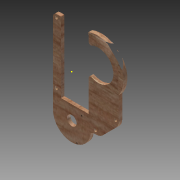
# Autodesk Inventor part: p1
Saved by Autodesk Inventor 2015 (Build 190159000, 159)
## iProperties
Created: 2016-02-03
Part Number: p1
Material: Generic
Document SubType Name: Modeling
Designer: david
Density: 1 g/cm^3
Appearance: Birch - Natural Polished
Author: david
Autodesk Inventor part; units mm, degrees
ref_plane "YZ Plane" through (0, 0, 0) normal (1, 0, 0) x (0, 1, 0)
ref_plane "XZ Plane" through (0, 0, 0) normal (0, 1, 0) x (-1, 0, 0)
ref_plane "XY Plane" through (0, 0, 0) normal (0, 0, 1) x (1, 0, 0)
sketch "Sketch1" plane through (0, 0, 0) normal (0, 1, 0) x (-1, 0, 0)
  line L0 (20, 45) -> (-20, 45)
  line L1 (-20, 45) -> (-20, -45)
  line L2 (-20, -45) -> (20, -45)
  line L3 (20, -45) -> (20, 45)
  line L4 (20, 45) -> (-20, -45) construction
  line L5 (-20, 45) -> (20, -45) construction
  arc A0 (-20, -45) -> (20, -45) centre (0, -45) ccw
  line L6 (20, -45) -> (20, -45)
  line L7 (20, -45) -> (20, 45)
  line L8 (20, 45) -> (20, 45)
  line L9 (20, 45) -> (20, -45)
  line L10 (-20, 45) -> (-50, 45)
  line L11 (-50, 45) -> (-50, -45)
  line L12 (-50, -45) -> (-20, -45)
  line L13 (-20, -45) -> (-20, 45)
  point P0 (0, 0)
  dimension "d0" = 40
  dimension "d1" = 90
  dimension "d7" = 0
  dimension "d8" = 90
  dimension "d35" = 30
  constraints: 28 end point, 6 equal length, 3 horizontal, 3 midpoint, 3 perpendicular, 2 point on circle, 1 centre point
  measures "d0" distance of L2.end L1.end
  measures "d1" distance of L1.end L0.end
  measures "d7" distance of L8.end L7.end
  measures "d8" distance of L7.end L6.end
  measures "d35" distance of L12.end L11.end
extrude "Extrusion1" add sketch "Sketch1" along normal blind 3.6
sketch "Sketch2" plane through (0, 3.6, 0) normal (0, 1, 0) x (1, 0, 0)
  arc A0 (20, 45) -> (-20, 45) centre (0, 45) ccw projected
  circle A1 centre (0, 45) radius 5.15
  point P0 (0, 0)
  dimension "d4" = 10.3
  constraints: 1 centre point, 1 coincident
  measures "d4" diameter of A1
extrude "Extrusion2" cut sketch "Sketch2" against normal blind 3.6
sketch "Sketch3" plane through (0, 0, 0) normal (0, -1, 0) x (1, 0, 0)
  line L0 (-20, 45) -> (50, 45) projected
  line L1 (-11.5, 45) -> (18, 45)
  line L2 (18, 45) -> (18, -30)
  line L3 (18, -30) -> (-11.5, -30)
  line L4 (-11.5, -30) -> (-11.5, 45)
  circle A0 centre (28, 20) radius 16.25
  line L5 (-20, -45) -> (-20, 45) projected
  line L6 (50, 45) -> (50, -45) projected
  point P0 (0, 0)
  point P1 (16, 45)
  dimension "d10" = 29.5
  dimension "d11" = 75
  dimension "d13" = 32.5
  dimension "d15" = 25
  dimension "d37" = 32
  dimension "d39" = 22
  constraints: 8 end point, 2 parallel, 1 centre point, 1 horizontal, 1 perpendicular, 1 point on line
  measures "d10" distance of L2.end L3.end
  measures "d11" distance of L1.end L2.end
  measures "d13" diameter of A0
  measures "d15" distance from line of L0 A0.centre
  measures "d37" distance between parallel lines of L6 L2
  measures "d39" distance from line of L6 A0.centre
extrude "Extrusion3" cut sketch "Sketch3" against normal blind 10
fillet "Fillet2" radius 2 3 edges at (18, 1.8, 45) (18, 1.8, 32.8087) (18, 1.8, 7.1913)
fillet "Fillet3" radius 4 3 edges at (50, 1.8, 45) (-20, 1.8, 45) (20, 1.8, -45)
chamfer "Chamfer1" distance 20 angle 45 1 edges at (50, 1.8, -45)
fillet "Fillet4" radius 10 2 edges at (30, 1.8, -45) (50, 1.8, -25)
sketch "Sketch6" plane through (3.0674, 0, -14.7029) normal (0, -1, 0) x (1, 0, 0)
  circle A0 centre (21.9326, -26.7971) radius 1.5
  circle A1 centre (43.4326, -6.7971) radius 1.5
  circle A2 centre (43.4326, 56.2029) radius 1.5
  line L0 (25.8579, -30.2971) -> (23.6643, -30.2971)
  line L1 (46.9326, 55.7029) -> (46.9326, -5.2971)
  line L2 (-23.0674, -30.2971) -> (-23.0674, 55.7029)
  line L3 (-16, 59.7029) -> (42.9326, 59.7029)
  circle A3 centre (18.4326, 43) radius 1.75
  line L4 (-23.0674, -30.2971) -> (-23.0674, 55.7029) projected
  line L5 (16.9326, 59.7029) -> (42.9326, 59.7029) projected
  line L6 (46.9326, 55.7029) -> (46.9326, -6.155) projected
  line L7 (22.7905, -30.2971) -> (20.5969, -30.2971) projected
  point P0 (0, 0)
  dimension "d56" = 3
  dimension "d53" = 3
  dimension "d50" = 3
  dimension "d58" = 3.5
  dimension "d55" = 3.5
  dimension "d57" = 25
  dimension "d54" = 20
  dimension "d52" = 3.5
  dimension "d51" = 3.5
  dimension "d45" = 3.5
  dimension "d46" = 25
  dimension "d62" = 0
  dimension "d63" = 0
  dimension "d64" = 0
  dimension "d65" = 0
  dimension "d66" = 0
  dimension "d67" = 0
  dimension "d68" = 25
  dimension "d69" = 0
  dimension "d70" = 0
  constraints: 8 end point, 4 centre point
  measures "d56" diameter of A0
  measures "d53" diameter of A1
  measures "d50" diameter of A2
  measures "d58" distance from line of L0 A0.centre
  measures "d55" distance from line of L1 A1.centre
  measures "d57" distance from line of L1 A0.centre
  measures "d54" vertical distance of A1.centre A0.centre
  measures "d52" distance from line of A2.centre L3
  measures "d51" distance from line of L1 A2.centre
  measures "d45" diameter of A3
  measures "d46" horizontal distance of A3.centre A2.centre
  measures "d62" distance between parallel lines of L2 L4
  measures "d63" distance of L4.end L2.end
  measures "d64" distance between parallel lines of L5 L3
  measures "d65" distance of L5.end L3.end
  measures "d66" distance between parallel lines of L6 L1
  measures "d67" distance of L6.start L1.start
  measures "d68" distance from line of L7 L1.end
  measures "d69" distance between parallel lines of L0 L7
  measures "d70" distance of L4.start L2.start
extrude "Extrusion6" cut sketch "Sketch6" against normal blind 10
sketch "Sketch7" plane through (33.0492, 0, -22.6689) normal (0, -1, 0) x (1, 0, 0)
  circle A0 centre (-49.5492, 64.1689) radius 1.5
  circle A1 centre (-49.5492, -0.8311) radius 1.5
  line L0 (-49.0492, 67.6689) -> (12.9508, 67.6689)
  line L1 (-53.0492, -23.8754) -> (-53.0492, 41)
  arc A2 (-53.0492, -23.8754) -> (-46.6341, -27.064) centre (-49.0492, -23.8754) ccw
  line L2 (-53.0492, -22.3311) -> (-53.0492, 63.6689) projected
  line L3 (-49.0492, 67.6689) -> (-44.5492, 67.6689) projected
  point P0 (0, 0)
  dimension "d74" = 3
  dimension "d71" = 3
  dimension "d76" = 3.5
  dimension "d75" = 3.5
  dimension "d73" = 3.5
  dimension "d72" = 65
  dimension "d80" = 0
  dimension "d81" = 0
  constraints: 4 end point, 3 centre point, 2 point on circle
  measures "d74" diameter of A0
  measures "d71" diameter of A1
  measures "d76" distance from line of L0 A0.centre
  measures "d75" distance from line of L1 A0.centre
  measures "d73" distance from line of L1 A1.centre
  measures "d72" distance of A1.centre A0.centre
  measures "d80" distance between parallel lines of L2 L1
  measures "d81" distance between parallel lines of L3 L0
extrude "Extrusion7" cut sketch "Sketch7" against normal blind 10
sketch "Sketch8" plane through (0, 0, 0) normal (0, -1, 0) x (1, 0, 0)
  point P0 (0, 0)
sketch "Sketch9" plane through (0, 3.6, 0) normal (0, 1, 0) x (1, 0, 0)
  line L0 (20, -45) -> (46, -45) projected
  line L1 (50, -41) -> (50, 20.8579) projected
  line L2 (18, -43) -> (18, -45.6174)
  arc A0 (18, -43) -> (20, -45) centre (20, -43) ccw projected
  arc A1 (18, -45.6174) -> (39.4564, -45) centre (28, -20) ccw
  arc A2 (50, -36.5) -> (50, -3.5) centre (28, -20) ccw
  point P0 (0, 0)
  dimension "d82" = 25
  dimension "d83" = 22
  constraints: 4 point on circle, 3 point on line, 2 centre point, 2 end point, 1 coincident, 1 tangent, 1 vertical
  measures "d82" distance from line of L0 point (28, -20)
  measures "d83" distance from line of point (28, -20) L1
extrude "Extrusion8" add sketch "Sketch9" against normal blind 3.6
fillet "Fillet5" radius 2 4 edges at (18, 1.8, 45.6174) (50, 1.8, 3.5) (50, 1.8, 36.5) (39.4564, 1.8, 45)
body "Solid1"
